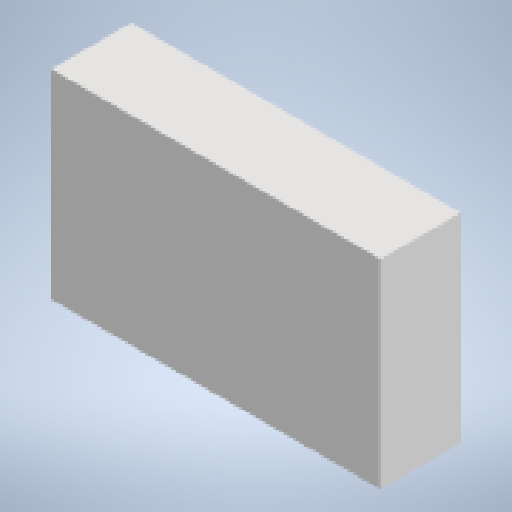
# Autodesk Inventor part: uMule-uchwyt_dx
Saved by Autodesk Inventor 2024.2 (Build 282272000, 272)
## iProperties
Created: 2024-10-21
Part Number: uMule-uchwyt_dx
Material: Ogólny
Document SubType Name: Modeling
Designer: owozn
Density: 1 g/cm^3
Appearance: Domyślna
Author: owozn
Autodesk Inventor part; units mm, degrees
ref_plane "YZ Plane" through (0, 0, 0) normal (1, 0, 0) x (0, 1, 0)
ref_plane "XZ Plane" through (0, 0, 0) normal (0, 1, 0) x (-1, 0, 0)
ref_plane "XY Plane" through (0, 0, 0) normal (0, 0, 1) x (1, 0, 0)
sketch "Szkic1" plane through (0, 0, 0) normal (0, 0, 1) x (1, 0, 0)
  line L0 (-28.7, 0) -> (28.7, 0) construction
  line L1 (0, -17.36) -> (0, 17.36) construction
  line L2 (-20.5, -12.4) -> (20.5, -12.4)
  line L3 (20.5, -12.4) -> (20.5, 12.4)
  line L4 (20.5, 12.4) -> (-20.5, 12.4)
  line L5 (-20.5, 12.4) -> (-20.5, -12.4)
  line L6 (-20.5, -12.4) -> (20.5, 12.4) construction
  line L7 (20.5, -12.4) -> (-20.5, 12.4) construction
  point P0 (0, 0)
  dimension "d0" = 41
  dimension "d1" = 24.8
  constraints: 12 end point, 2 midpoint, 2 parallel, 1 horizontal, 1 perpendicular
  measures "d0" distance of L4.end L3.end
  measures "d1" distance of L3.end L2.end
extrude "Wyciągnięcie proste1" add sketch "Szkic1" along normal blind 10
sketch "Szkic2" plane through (-20.5, -12.4, 0) normal (0, -1, 0) x (1, 0, 0)
  point P0 (20.5, 0)
